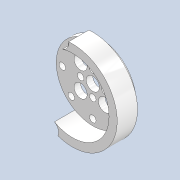
# Autodesk Inventor part: s_base6
Saved by Autodesk Inventor 2022 (Build 260153000, 153)
## iProperties
Created: 2021-08-27
Part Number: s_base6
Material: ABS プラスチック
Document SubType Name: Modeling
Designer: Yuta Kage
Density: 1.06 g/cm^3
Appearance: 滑らか - 白
Author: Yuta Kage
Autodesk Inventor part; units mm, degrees
ref_plane "YZ Plane" through (0, 0, 0) normal (1, 0, 0) x (0, 1, 0)
ref_plane "XZ Plane" through (0, 0, 0) normal (0, 1, 0) x (-1, 0, 0)
ref_plane "XY Plane" through (0, 0, 0) normal (0, 0, 1) x (1, 0, 0)
sketch "スケッチ1" plane through (0, 0, 0) normal (0, 0, 1) x (1, 0, 0)
  circle A0 centre (0, 0) radius 18
  dimension "d0" = 36
  constraints: 1 centre point, 1 coincident
  measures "d0" diameter of A0
extrude "押し出し1" add sketch "スケッチ1" along normal blind 3.25
sketch "スケッチ2" plane through (0, 0, 3.25) normal (0, 0, 1) x (1, 0, 0)
  circle A0 centre (0, 0) radius 6
  point P0 (0, 6)
  point P1 (-6, 0)
  point P2 (0, -6)
  point P3 (6, 0)
  dimension "d3" = 12
  dimension "d6" = 360
  constraints: 1 coincident, 1 vertical alignment, 7 other
hole "穴1" at (0, 6, 3.25) at (-6, 0, 3.25) at (0, -6, 3.25) at (6, 0, 3.25) direction (0, 0, -1) diameter 3.2 end through all clearance for "Socket Head Cap Screw" size "M3" standard "Ansi Metric M Profile"
sketch "スケッチ3" plane through (0, 0, 0) normal (0, 0, -1) x (-1, 0, 0)
  circle A0 centre (0, 0) radius 8.5
  point P0 (-6.0104, 6.0104)
  point P1 (-6.0104, -6.0104)
  point P2 (6.0104, -6.0104)
  point P3 (6.0104, 6.0104)
  dimension "d15" = 17
  dimension "d18" = 360
  constraints: 1 coincident, 1 horizontal alignment, 8 other
hole "穴2" at (6.0104, 6.0104, 0) at (6.0104, -6.0104, 0) at (-6.0104, -6.0104, 0) at (-6.0104, 6.0104, 0) direction (0, 0, 1) diameter 3.2 end through all counterbore diameter 6.5 counterbore depth 10 clearance for "Socket Head Cap Screw" size "M3" standard "Ansi Metric M Profile"
sketch "スケッチ4" plane through (0, 0, 0) normal (0, 0, -1) x (-1, 0, 0)
  circle A0 centre (0, 0) radius 3.25
  dimension "d27" = 6.5
  constraints: 1 centre point, 1 coincident
  measures "d27" diameter of A0
extrude "押し出し2" cut sketch "スケッチ4" against normal blind 8
sketch "スケッチ5" plane through (0, 0, 3.25) normal (0, 0, 1) x (1, 0, 0)
  circle A0 centre (0, 0) radius 15
  point P0 (0, -15)
  point P1 (10.6066, -10.6066)
  point P2 (15, 0)
  point P3 (10.6066, 10.6066)
  point P4 (0, 15)
  point P5 (-10.6066, 10.6066)
  point P6 (-15, 0)
  point P7 (-10.6066, -10.6066)
  dimension "d31" = 30
  dimension "d34" = 360
  constraints: 1 coincident, 1 vertical alignment, 11 other
hole "穴3" at (0, -15, 3.25) at (10.6066, -10.6066, 3.25) at (15, 0, 3.25) at (10.6066, 10.6066, 3.25) at (0, 15, 3.25) at (-10.6066, 10.6066, 3.25) at (-15, 0, 3.25) at (-10.6066, -10.6066, 3.25) direction (0, 0, -1) diameter 3.2 end through all clearance for "Socket Head Cap Screw" size "M3" standard "Ansi Metric M Profile"
sketch "スケッチ7" plane through (0, 0, 3.25) normal (0, 0, 1) x (1, 0, 0)
  circle A0 centre (2.0753, 21.9019) radius 4
  circle A1 centre (-17, 14) radius 4 construction
  circle A2 centre (-3.264, -21.7565) radius 4
  circle A3 centre (0, 0) radius 18
  line L0 (-3.264, -21.7565) -> (0, 0) construction
  circle A4 centre (-20.8592, 6.9924) radius 4 construction
  circle A5 centre (-10.8624, 19.1313) radius 4 construction
  line L1 (-10.8624, 19.1313) -> (0, 0) construction
  line L2 (0, 0) -> (-20.8592, 6.9924) construction
  line L3 (0, 0) -> (2.0753, 21.9019) construction
  arc A6 (-3.8575, -25.7123) -> (2.4526, 25.8841) centre (0, 0) ccw
  circle A7 centre (0, 0) radius 18
  circle A8 centre (-5.8935, 21.1959) radius 4
  circle A9 centre (-10.8278, -19.1509) radius 4
  circle A10 centre (0, 0) radius 22
  point P0 (-1.9091, 21.5489)
  point P1 (-7.1494, -20.8059)
  point P2 (-4.822, 17.3421)
  point P3 (-8.8591, -15.669)
  point P4 (-7.0459, -20.4537)
  point P5 (-1.9247, 21.9156)
  point P6 (-1.9091, 21.5489)
  dimension "d57" = 44
  dimension "d46" = 17
  dimension "d47" = 14
  dimension "d48" = 8
  dimension "d49" = 8
  dimension "d50" = 8
  dimension "d51" = 8
  dimension "d52" = 8
  dimension "d53" = 35
  dimension "d54" = 100
  dimension "d55" = 8
  dimension "d56" = 8
  constraints: 11 tangent, 10 centre point, 8 end point, 6 point on circle, 3 coincident, 1 point on line, 3 other
  measures "d46" horizontal distance of A1.centre point (0, 0)
  measures "d47" vertical distance of point (0, 0) A1.centre
  measures "d48" diameter of A1
  measures "d49" diameter of A0
  measures "d50" diameter of A2
  measures "d51" diameter of A4
  measures "d52" diameter of A5
  measures "d53" angle of L1 L3
  measures "d54" angle of L2 L0
  measures "d55" diameter of A8
  measures "d56" diameter of A9
extrude "押し出し4" add sketch "スケッチ7" against normal up to surface (3.25 mm away) contours A10 A2 A3 A0 | A0 A10 | A3 A8 A0 | A2 A10 | A9 A3 A2 picked at (1.947, 20.5476) picked at (-3.0622, -20.4112)
